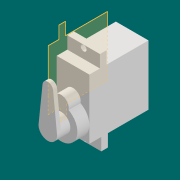
# Autodesk Inventor part: Servo
Saved by Autodesk Inventor 2020.1 (Build 241239000, 239)
## iProperties
Created: 2020-01-27
Part Number: Servo
Material: Generic
Document SubType Name: Modeling
Designer: Pluscrafter
Density: 1 g/cm^3
Appearance: Default
Author: Pluscrafter
Autodesk Inventor part; units mm, degrees
ref_plane "YZ Plane" through (0, 0, 0) normal (1, 0, 0) x (0, 1, 0)
ref_plane "XZ Plane" through (0, 0, 0) normal (0, 1, 0) x (-1, 0, 0)
ref_plane "XY Plane" through (0, 0, 0) normal (0, 0, 1) x (1, 0, 0)
sketch "Sketch1" plane through (0, 0, 0) normal (0, 0, 1) x (1, 0, 0)
  line L0 (0, 0) -> (12.3, 0)
  line L1 (12.3, 0) -> (12.3, 22.6)
  line L2 (12.3, 22.6) -> (0, 22.6)
  line L3 (0, 22.6) -> (0, 0)
  line L4 (6.15, 22.6) -> (6.15, 0) construction
  arc A0 (3.3318, 11.6163) -> (8.9682, 11.6163) centre (6.15, 6.15) ccw
  arc A1 (8.9682, 11.6163) -> (3.3318, 11.6163) centre (6.15, 12.3) ccw
  dimension "d0" = 12.3
  dimension "d1" = 22.6
  dimension "d2" = 6.15
  dimension "d3" = 6.15
  dimension "d4" = 5.8
  constraints: 10 end point, 4 point on circle, 2 centre point, 2 midpoint, 2 parallel, 2 point on line, 1 coincident, 1 horizontal, 1 perpendicular, 1 tangent
  measures "d0" distance of L2.end L1.end
  measures "d1" distance of L0.end L1.end
  measures "d2" distance from line of point (6.15, 6.15) L0
  measures "d3" distance from line of L1 point (6.15, 6.15)
  measures "d4" diameter of A1
extrude "Extrusion1" add sketch "Sketch1" against normal blind 22.3
sketch "Sketch2" plane through (0, 0, 0) normal (0, 0, 1) x (1, 0, 0)
  line L0 (0, 0) -> (12.3, 0)
  line L1 (12.3, 0) -> (12.3, 22.6)
  line L2 (12.3, 22.6) -> (0, 22.6)
  line L3 (0, 22.6) -> (0, 0)
  line L4 (6.15, 22.6) -> (6.15, 0) construction
  arc A0 (3.3318, 11.6163) -> (8.9682, 11.6163) centre (6.15, 6.15) ccw
  arc A1 (8.9682, 11.6163) -> (3.3318, 11.6163) centre (6.15, 12.3) ccw
  dimension "d7" = 12.3
  dimension "d8" = 22.6
  dimension "d9" = 6.15
  dimension "d10" = 6.15
  dimension "d11" = 5.8
  constraints: 10 end point, 4 point on circle, 2 centre point, 2 midpoint, 2 parallel, 2 point on line, 1 coincident, 1 horizontal, 1 perpendicular, 1 tangent
  measures "d7" distance of L2.end L1.end
  measures "d8" distance of L0.end L1.end
  measures "d9" distance from line of point (6.15, 6.15) L0
  measures "d10" distance from line of L1 point (6.15, 6.15)
  measures "d11" diameter of A1
extrude "Extrusion2" add sketch "Sketch2" along normal blind 4.5 contours A0 A1
sketch "Sketch3" plane through (0, 22.6, 0) normal (0, 1, 0) x (1, 0, 0)
  line L0 (12.3, 0) -> (0, 0) construction
  line L1 (12.3, 0) -> (12.3, 22.3) construction
  line L2 (0, 0) -> (0, 22.3) construction
  line L3 (12.3, 4) -> (0, 4)
  line L4 (0, 4) -> (0, 6.5)
  line L5 (0, 6.5) -> (12.3, 6.5)
  line L6 (12.3, 6.5) -> (12.3, 4)
  dimension "d14" = 4
  dimension "d15" = 2.5
  constraints: 8 end point, 2 parallel, 2 point on line, 1 horizontal, 1 perpendicular
  measures "d14" distance between parallel lines of L0 L3
  measures "d15" distance between parallel lines of L5 L3
extrude "Extrusion3" add sketch "Sketch3" along normal blind 4.7
sketch "Sketch4" plane through (0, 0, -22.3) normal (0, -1, 0) x (1, 0, 0)
  line L0 (12.3, 15.3) -> (0, 15.3)
  line L1 (0, 15.3) -> (0, 17.8)
  line L2 (0, 17.8) -> (12.3, 17.8)
  line L3 (12.3, 17.8) -> (12.3, 15.3)
  line L4 (0, 22.3) -> (6.15, 22.3) construction
  line L5 (0, 22.3) -> (0, 0) construction
  line L6 (12.3, 0) -> (0, 0) construction
  line L7 (12.3, 22.3) -> (12.3, 0) construction
  line L8 (6.15, 22.3) -> (12.3, 22.3) construction
  dimension "d19" = 2.5
  dimension "d20" = 4.5
  constraints: 8 end point, 2 parallel, 1 horizontal, 1 perpendicular
  measures "d19" distance between parallel lines of L2 L0
  measures "d20" distance between parallel lines of L8 L2
extrude "Extrusion4" add sketch "Sketch4" along normal blind 4.7
sketch "Sketch5" plane through (0, 22.6, -4) normal (0, 0, 1) x (1, 0, 0)
  line L0 (12.3, 0) -> (0, 0) construction
  line L1 (12.3, 0) -> (12.3, 4.7) construction
  line L2 (0, 4.7) -> (12.3, 4.7) construction
  line L3 (0, 0) -> (0, 4.7) construction
  line L4 (0, 4.7) -> (12.3, 4.7) projected
  line L5 (6.15, 4.7) -> (6.15, 0)
  circle A0 centre (6.15, 3.6) radius 1.1
  point P0 (0, -22.6)
  dimension "d23" = 1.1
  constraints: 2 end point, 2 midpoint, 1 coincident, 1 point on line, 1 vertical alignment, 2 other
  measures "d23" distance from line of L2 point (6.15, 3.6)
extrude "Extrusion5" cut sketch "Sketch5" against normal blind 10
sketch "Sketch6" plane through (0, 0, -4.5) normal (0, 0, 1) x (1, 0, 0)
  line L0 (0, 0) -> (12.3, 0) construction
  line L1 (0, 0) -> (0, -4.7) construction
  line L2 (12.3, -4.7) -> (0, -4.7) construction
  line L3 (12.3, 0) -> (12.3, -4.7) construction
  line L4 (0, -4.7) -> (12.3, -4.7) construction
  line L5 (6.15, -4.7) -> (6.15, 0) construction
  line L6 (12.3, 0) -> (0, 0) construction
  circle A0 centre (6.15, -3.6) radius 1.1
  dimension "d26" = 1.1
  constraints: 2 end point, 2 midpoint, 1 coincident, 1 point on line, 1 vertical alignment, 2 other
  measures "d26" distance from line of L2 point (6.15, -3.6)
extrude "Extrusion6" cut sketch "Sketch6" against normal blind 10
sketch "Sketch7" plane through (0, 0, 4.5) normal (0, 0, 1) x (1, 0, 0)
  arc A0 (3.3318, 11.6163) -> (8.9682, 11.6163) centre (6.15, 6.15) ccw projected
  arc A1 (8.9682, 11.6163) -> (3.3318, 11.6163) centre (6.15, 12.3) ccw projected
  circle A2 centre (6.15, 6.15) radius 3.5
  point P0 (0, 0)
  dimension "d29" = 7
  constraints: 1 centre point, 1 coincident
  measures "d29" diameter of A2
extrude "Extrusion7" add sketch "Sketch7" along normal blind 5 contours A2
sketch "Sketch8" plane through (6.15, 6.15, 9.5) normal (0, 0, 1) x (1, 0, 0)
  circle A0 centre (0, 0) radius 3.5 construction
  line L0 (0, 0) -> (0, 13.1535)
  circle A1 centre (0, 0) radius 3.5 construction
  arc A2 (1.9885, 14.0145) -> (-1.9885, 14.0145) centre (0, 13.8) ccw
  line L1 (-3.5, 0) -> (-1.9885, 14.0145)
  line L2 (3.5, 0) -> (1.9885, 14.0145)
  line L3 (0, -12.2559) -> (0, 3.5)
  line L4 (0, 15.8) -> (0, 18.1002)
  line L5 (3.5, 0) -> (-3.5, 0)
  point P0 (-6.15, -6.15)
  point P1 (0, -3.5)
  dimension "d32" = 19.3
  dimension "d33" = 2
  constraints: 12 end point, 7 point on circle, 2 point on line, 2 tangent, 2 vertical, 1 centre point, 1 coincident
  measures "d32" distance of L4.start A1.start
  measures "d33" distance of point (0, 13.8) L4.start
extrude "Extrusion8" add sketch "Sketch8" against normal blind 1.5
body "Solid1"
